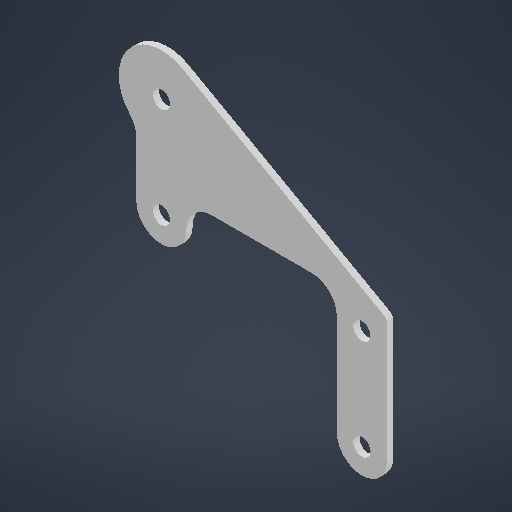
# Autodesk Inventor part: topFrontCorners
Saved by Autodesk Inventor 2025.1 (Build 291241000, 241)
## iProperties
Created: 2025-01-10
Part Number: topFrontCorners
Material: Generic
Document SubType Name: Modeling
Designer: Jahan
Density: 1 g/cm^3
Appearance: Default
Author: Jahan
Autodesk Inventor part; units mm, degrees
ref_plane "YZ Plane" through (0, 0, 0) normal (1, 0, 0) x (0, 1, 0)
ref_plane "XZ Plane" through (0, 0, 0) normal (0, 1, 0) x (-1, 0, 0)
ref_plane "XY Plane" through (0, 0, 0) normal (0, 0, 1) x (1, 0, 0)
sketch "Sketch1" plane through (0, 0, 0) normal (0, 0, 1) x (1, 0, 0)
  circle A0 centre (-29.4482, 25.881) radius 2.1844
  circle A1 centre (-29.4482, 0.481) radius 2.1844
  circle A2 centre (21.3518, 0.481) radius 2.1844
  circle A3 centre (21.3518, -24.919) radius 2.1844
  line L0 (26.6858, 6.831) -> (-24.1755, 35.3007)
  arc A4 (27.7018, 5.815) -> (26.6858, 6.831) centre (25.394, 4.5232) ccw
  line L1 (27.7018, 5.815) -> (27.7018, -24.919)
  line L2 (15.0018, -24.919) -> (46.7518, -24.919) construction
  arc A5 (-35.8023, 0.481) -> (-23.0942, 0.481) centre (-29.4482, 0.481) ccw
  line L3 (-23.0942, 0.481) -> (-23.0942, 6.831)
  arc A6 (15.0018, -24.919) -> (27.7018, -24.919) centre (21.3518, -24.919) ccw
  arc A7 (-35.8023, 14.3676) -> (-37.4471, 18.6319) centre (-42.1523, 14.3676) ccw
  line L4 (-35.8023, 14.3676) -> (-35.8023, 0.481)
  arc A8 (-24.1755, 35.3007) -> (-37.4471, 18.6319) centre (-29.4482, 25.881) ccw
  arc A9 (-16.7482, 6.831) -> (-23.0942, 0.708) centre (-16.7482, 0.481) ccw
  arc A10 (15.0018, 0.481) -> (8.6518, 6.831) centre (8.6518, 0.481) ccw
  line L5 (8.6518, 6.831) -> (-16.7482, 6.831)
  line L6 (15.0018, 0.481) -> (15.0018, -24.919)
  point P0 (0, 0)
  dimension "d0" = 6.35
  dimension "d1" = 6.35
  constraints: 14 end point, 14 point on circle, 11 centre point, 5 tangent, 2 coincident, 2 horizontal, 2 point on line, 2 vertical, 1 perpendicular
  measures "d0" radius of A7
  measures "d1" radius of A9
extrude "Extrusion1" add sketch "Sketch1" along normal blind 1.5875
body "Solid1"
